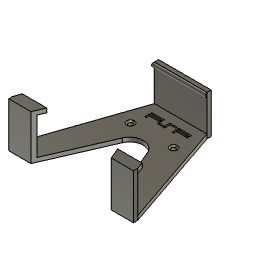
Sony PSP 1000 (Autodesk Fusion 360 design; units mm, degrees)
Autodesk Fusion 360 part; units mm, degrees
sketch "Top" plane through (0, 0, 0) normal (0, 0, 1) x (1, 0, 0)
  line L0 (59.2894, -12.484) -> (59.2841, -12.484)
  line L1 (59.2841, -12.484) -> (59.2841, -12.4898)
  line L2 (59.2841, -12.4898) -> (51.2779, -12.4898)
  line L3 (51.2779, -12.4898) -> (51.2779, -14.4245)
  line L4 (51.2779, -14.4245) -> (50.2771, -14.4245)
  line L5 (50.2771, -14.4245) -> (50.2771, -11.4736)
  line L6 (50.2771, -11.4736) -> (50.4315, -11.4736)
  line L7 (50.4315, -11.4736) -> (50.4315, -11.4723)
  line L8 (50.4315, -11.4723) -> (58.2887, -11.5)
  line L9 (58.2887, -11.5) -> (58.283, -10.5632)
  line L10 (58.283, -10.5632) -> (50.2771, -10.5355)
  line L11 (50.2771, -10.5355) -> (50.2828, -9.5486)
  line L12 (50.2828, -9.5486) -> (59.2837, -9.5486)
  line L13 (59.2837, -9.5486) -> (59.2837, -9.565)
  line L14 (59.2837, -9.565) -> (59.2894, -9.565)
  line L15 (59.2894, -9.565) -> (59.2894, -12.484)
  line L16 (49.1011, -10.5494) -> (44.8406, -10.5786)
  line L17 (44.8406, -10.5786) -> (44.8406, -14.4537)
  line L18 (44.8406, -14.4537) -> (39.5795, -14.4245)
  line L19 (39.5795, -14.4245) -> (39.5795, -13.4237)
  line L20 (39.5795, -13.4237) -> (43.8385, -13.4237)
  line L21 (43.8385, -13.4237) -> (43.8413, -9.5486)
  line L22 (43.8413, -9.5486) -> (49.1011, -9.5486)
  line L23 (49.1011, -9.5486) -> (49.1011, -10.5494)
  line L24 (31.7113, -12.5044) -> (31.7113, -14.4245)
  line L25 (31.7113, -14.4245) -> (30.7106, -14.4245)
  line L26 (30.7106, -14.4245) -> (30.7106, -11.5015)
  line L27 (30.7106, -11.5015) -> (30.8648, -11.5015)
  line L28 (30.8648, -11.5015) -> (30.8648, -11.5001)
  line L29 (30.8648, -11.5001) -> (38.7247, -11.4943)
  line L30 (38.7247, -11.4943) -> (38.7192, -10.5436)
  line L31 (38.7192, -10.5436) -> (30.7106, -10.5494)
  line L32 (30.7106, -10.5494) -> (30.7161, -9.5486)
  line L33 (30.7161, -9.5486) -> (39.7172, -9.5486)
  line L34 (39.7172, -9.5486) -> (39.7172, -9.565)
  line L35 (39.7172, -9.565) -> (39.7227, -9.565)
  line L36 (39.7227, -9.565) -> (39.7227, -12.4987)
  line L37 (39.7227, -12.4987) -> (39.7172, -12.4987)
  line L38 (39.7172, -12.4987) -> (39.7172, -12.5044)
  line L39 (39.7172, -12.5044) -> (31.7113, -12.5044)
  line L40 (64, -3) -> (64, 0)
  line L41 (64, 0) -> (26, 0)
  line L42 (26, 0) -> (26, -3)
  line L43 (26, -3) -> (0, -79)
  line L44 (0, -79) -> (0, -82)
  line L45 (0, -82) -> (16, -82)
  line L46 (16, -82) -> (35.8941, -36.045)
  spline S0 degree 3 poles (35.8941, -36.045) (39.3461, -28.0709) (50.6539, -28.0709) (54.106, -36.045) knots 7 7 7 7 8 8 8 8
  line L47 (54.106, -36.045) -> (74, -82)
  line L48 (74, -82) -> (90, -82)
  line L49 (90, -82) -> (90, -79)
  line L50 (90, -79) -> (64, -3)
extrude "Extrude1" add sketch "Top" along normal blind 32.47
sketch "Side" plane through (0, 0, 0) normal (1, 0, 0) x (0, 1, 0)
  line L0 (-82, 37.505) -> (-82, 32.4661)
  line L1 (-82, 32.4661) -> (-74, 32.4661)
  line L2 (-74, 32.4661) -> (-74, 29.4661)
  line L3 (-74, 29.4661) -> (-79, 29.4661)
  line L4 (-79, 29.4661) -> (-79, 2.9661)
  line L5 (-79, 2.9661) -> (-3, 2.9661)
  line L6 (-3, 2.9661) -> (-3, 25.9661)
  spline S0 degree 3 poles (-3, 25.9661) (-3.8284, 25.9661) (-4.5, 26.6377) (-4.5, 27.4661) (-4.5, 28.2945) (-3.8284, 28.9661) (-3, 28.9661) knots 7 7 7 7 8 8 8 9 9 9 9
  line L7 (-3, 28.9661) -> (0, 28.9661)
  line L8 (0, 28.9661) -> (0, 37.505)
  line L9 (0, 37.505) -> (-82, 37.505)
extrude "Extrude2" cut sketch "Side" along normal blind 90
hole "Hole1" at (29.5044, -23.6505, 2.9661) direction (0, 0, -1) diameter 3.5 depth 3 tip angle 118 countersink diameter 5.5 countersink angle 90
hole "Hole2" at (60.4957, -23.6505, 2.9661) direction (0, 0, -1) diameter 3.5 depth 3 tip angle 118 countersink diameter 5.5 countersink angle 90
